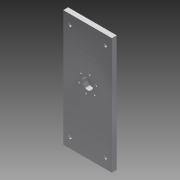
# Autodesk Inventor part: Part74
Saved by Autodesk Inventor 2015 (Build 190159000, 159)
## iProperties
Created: 2015-01-10
Part Number: Part74
Material: Generic
Document SubType Name: Modeling
Designer: mastkee16
Density: 1 g/cm^3
Appearance: Aluminum - Polished
Author: mastkee16
Autodesk Inventor part; units mm, degrees
ref_plane "YZ Plane" through (0, 0, 0) normal (1, 0, 0) x (0, 1, 0)
ref_plane "XZ Plane" through (0, 0, 0) normal (0, 1, 0) x (-1, 0, 0)
ref_plane "XY Plane" through (0, 0, 0) normal (0, 0, 1) x (1, 0, 0)
sketch "Sketch1" plane through (0, 0, 0) normal (0, 0, 1) x (1, 0, 0)
  point P0 (0, 0)
sketch "Sketch2" plane through (0, 0, 0) normal (0, 0, 1) x (1, 0, 0)
  line L0 (0, 0) -> (127, 0)
  line L1 (127, 0) -> (127, 304.8)
  line L2 (127, 304.8) -> (0, 304.8)
  line L3 (0, 304.8) -> (0, 0)
  circle A0 centre (17.338, 279.4) radius 3.9687
  circle A1 centre (109.662, 279.4) radius 3.9687
  circle A2 centre (17.338, 25.4) radius 3.9688
  circle A3 centre (109.662, 25.4) radius 3.9688
  dimension "d0" = 127
  dimension "d1" = 304.8
  dimension "d2" = 7.9375
  dimension "d3" = 25.4
  dimension "d4" = 17.338
  dimension "d5" = 7.9375
  dimension "d6" = 17.338
  dimension "d7" = 25.4
  dimension "d8" = 7.9375
  dimension "d9" = 17.338
  dimension "d10" = 25.4
  dimension "d11" = 7.9375
  dimension "d12" = 17.338
  dimension "d13" = 25.4
  constraints: 8 end point, 4 centre point, 2 parallel, 1 horizontal, 1 perpendicular
  measures "d0" distance of L2.end L1.end
  measures "d1" distance of L1.end L0.end
  measures "d2" diameter of A0
  measures "d3" distance from line of A0.centre L2
  measures "d4" distance from line of L3 A0.centre
  measures "d5" diameter of A1
  measures "d6" distance from line of L1 A1.centre
  measures "d7" distance from line of L2 A1.centre
  measures "d8" diameter of A2
  measures "d9" distance from line of L3 A2.centre
  measures "d10" distance from line of L0 A2.centre
  measures "d11" diameter of A3
  measures "d12" distance from line of L1 A3.centre
  measures "d13" distance from line of L0 A3.centre
extrude "Extrusion1" add sketch "Sketch2" along normal blind 12.7
sketch "Sketch3" plane through (0, 0, 12.7) normal (0, 0, 1) x (1, 0, 0)
  line L0 (127, 304.8) -> (0, 304.8) projected
  line L1 (0, 0) -> (127, 0) projected
  line L2 (0, 304.8) -> (0, 0) projected
  line L3 (127, 0) -> (127, 304.8) projected
  circle A0 centre (46, 232.918) radius 0.635
  circle A1 centre (63.5, 250.4307) radius 0.635
  circle A2 centre (63.5, 215.4307) radius 0.635
  circle A3 centre (81, 232.918) radius 0.635
  circle A4 centre (63.5, 169.4307) radius 14.2875
  circle A5 centre (63.5, 169.4307) radius 23.8252
  point P0 (63.5, 232.9307)
  point P1 (68.244, 192.7788)
  point P2 (45.652, 185.2132)
  point P3 (40.9079, 161.8651)
  point P4 (58.756, 146.0826)
  point P5 (81.348, 153.6482)
  point P6 (86.0921, 176.9963)
  dimension "d18" = 63.5
  dimension "d19" = 63.5
  dimension "d31" = 1.27
  dimension "d32" = 1.27
  dimension "d33" = 1.27
  dimension "d34" = 1.27
  dimension "d45" = 34.9999
  dimension "d46" = 17.5
  dimension "d47" = 17.5
  dimension "d48" = 17.5
  dimension "d49" = 28.575
  dimension "d50" = 169.4307
  dimension "d53" = 23.8252
  dimension "d56" = 360
  dimension "d66" = 63.5
  dimension "d67" = 63.5
  dimension "d68" = 63.5
  dimension "d69" = 63.5
  dimension "d70" = 71.8693
  dimension "d71" = 71.882
  dimension "d72" = 71.882
  constraints: 5 centre point, 5 coincident, 10 other
  measures "d18" distance from line of L2 point (63.5, 232.931)
  measures "d19" distance from line of L3 point (63.5, 232.931)
  measures "d31" diameter of A0
  measures "d32" diameter of A1
  measures "d33" diameter of A2
  measures "d34" diameter of A3
  measures "d45" distance of point (63.5, 215.431) point (63.5, 250.431)
  measures "d46" distance of point (63.5, 232.931) point (63.5, 250.431)
  measures "d47" distance of point (63.5, 232.931) point (81, 232.918)
  measures "d48" distance of point (63.5, 232.931) point (46, 232.918)
  measures "d49" diameter of A4
  measures "d50" distance from line of L1 A4.centre
  measures "d53" distance of point (68.244, 192.779) A4.centre
  measures "d66" distance from line of L2 A4.centre
  measures "d67" distance of A4.centre point (63.5, 232.931)
  measures "d68" distance from line of L2 A1.centre
  measures "d69" distance from line of L2 A2.centre
  measures "d70" distance from line of L0 point (63.5, 232.931)
  measures "d71" distance from line of L0 point (46, 232.918)
  measures "d72" distance from line of L0 A3.centre
hole "Hole1" at (63.5, 232.9307, 12.7) direction (0, 0, -1) diameter 1.27 end through all
extrude "Extrusion2" cut sketch "Sketch3" against normal blind 25.4 contours A0 | A1 | A2 | A3
extrude "Extrusion3" cut sketch "Sketch3" against normal blind 25.4 contours A4
hole "Hole2" at (68.244, 192.7788, 12.7) at (45.652, 185.2132, 12.7) at (40.9079, 161.8651, 12.7) at (58.756, 146.0826, 12.7) at (81.348, 153.6482, 12.7) at (86.0921, 176.9963, 12.7) direction (0, 0, -1) diameter 5.08 end through all
body "Solid1"
